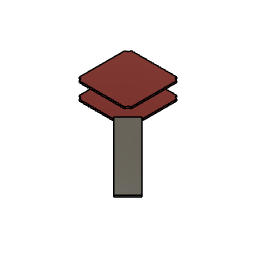
Drone+CAD (Autodesk Fusion 360 design; units mm, degrees)
Autodesk Fusion 360 part; units mm, degrees
sketch "Sketch1" plane through (0, 0, 0) normal (0, 0, 1) x (1, 0, 0)
  line L0 (0, 0) -> (165.1, 0)
  line L1 (165.1, 0) -> (165.1, 165.7389)
  line L2 (165.1, 165.7389) -> (0, 165.7389)
  line L3 (0, 165.7389) -> (0, 0)
  dimension "d1" = 165.1
  constraint horizontal L0
  constraint vertical L1
  constraint horizontal L2
  constraint vertical L3
  constraint coincident L0.start L3.end
  measures "d1" distance of L0.start L0.end
extrude "Extrude1" add sketch "Sketch1" along normal blind 5.08 makes body 1
hole "Hole1" at (0, 0, 5.08) direction (0, 0, -1) diameter 20.32 depth 20.32 tip angle 118 bodies 1
hole "Hole2" at (165.201, -0.1225, 5.08) direction (0, 0, -1) diameter 20.32 depth 20.32 tip angle 118 bodies 1
hole "Hole3" at (164.9404, 165.572, 5.08) direction (0, 0, -1) diameter 20.32 depth 12.7 tip angle 118 bodies 1
hole "Hole4" at (-0.0078, 165.2513, 5.08) direction (0, 0, -1) diameter 20.32 depth 12.7 tip angle 118 bodies 1
copy_body "CopyPasteBodies2" bodies 1 makes body 2
move_body "Move1" bodies 2 to x (1, 0, 0) y (0, 1, 0) z (0, 0, 1) at (0, 0, 50.8)
sketch "Sketch2" plane through (0, 0, 0) normal (0, 0, 1) x (1, 0, 0)
  line L0 (0, 0) -> (304.8, 0)
  line L1 (304.8, 0) -> (304.8, 63.5)
  line L2 (304.8, 63.5) -> (0, 63.5)
  line L3 (0, 63.5) -> (0, 0)
  dimension "d16" = 304.8
  dimension "d17" = 63.5
  constraint horizontal L0
  constraint vertical L1
  constraint horizontal L2
  constraint vertical L3
  constraint coincident L0.start L3.end
  measures "d16" distance of L0.start L0.end
  measures "d17" distance of L0.start L2.end
extrude "Extrude2" add sketch "Sketch2" along normal blind 5.08 separate body makes body 3
move_body "Move2" bodies 3 to x (1, 0, 0) y (0, 1, 0) z (0, 0, 1) at (22.8628, -100.7836, 8.488)
move_body "Move3" bodies 3 to x (0.707107, -0.707107, 0) y (0.707107, 0.707107, 0) z (0, 0, 1) at (174.8539, 87.9398, -3.2125)
named bodies: "Base 1", "Base 2"
